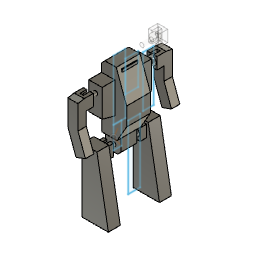
robo v3 (Autodesk Fusion 360 design; units mm, degrees)
Autodesk Fusion 360 part; units mm, degrees
note: some values were not read from the file. Set by a fixed rule: which face or edge a step refers to.
sketch "スケッチ1" plane through (0, 0, 0) normal (1, 0, 0) x (0, 1, 0) in component "球形ジョイント v1"
  circle A0 centre (0, 0) radius 2.5
  line L0 (3.5, -3.5) -> (-3.5, -3.5)
  line L1 (-3.5, -3.5) -> (-3.5, 3.5)
  line L2 (-3.5, 3.5) -> (3.5, 3.5)
  line L3 (3.5, 3.5) -> (3.5, -3.5)
  line L4 (3.5, -3.5) -> (-3.5, 3.5) construction
  line L5 (-3.5, -3.5) -> (3.5, 3.5) construction
  line L6 (4.5, -3.5) -> (2.5, -3.5)
  line L7 (2.5, -3.5) -> (2.5, 3.5)
  line L8 (2.5, 3.5) -> (4.5, 3.5)
  line L9 (4.5, 3.5) -> (4.5, -3.5)
  line L10 (4.5, -3.5) -> (2.5, 3.5) construction
  line L11 (2.5, -3.5) -> (4.5, 3.5) construction
  line L12 (2.5, 3.5) -> (2.5, 3.8624)
  line L13 (2.5, 3.8624) -> (-1, 3.8624)
  line L14 (-1, 3.8624) -> (-1, -3.5)
  point P0 (3.5, 0)
  dimension "d1" = 5
  dimension "d4" = 7
  dimension "d5" = 7
  dimension "d8" = 2
  dimension "d9" = 7
  dimension "d12" = 3.5
  constraint coincident A0.centre origin
  constraint horizontal L0
  constraint perpendicular L0 L1
  constraint parallel L0 L2
  constraint parallel L1 L3
  constraint coincident L4 A0.centre
  constraint coincident L5 A0.centre
  constraint horizontal L6
  constraint perpendicular L6 L7
  constraint parallel L6 L8
  constraint parallel L7 L9
  constraint coincident L10 P0
  constraint coincident L11 P0
  constraint midpoint L3 P0
  constraint perpendicular L8 L12
  constraint perpendicular L12 L13
  constraint coincident L0 L14.end
  constraint perpendicular L0 L14
  measures "d1" diameter of A0
  measures "d4" distance of L1.end L2.end
  measures "d5" distance of L0.end L1.end
  measures "d8" distance of L7.end L8.end
  measures "d9" distance of L6.end L7.end
  measures "d12" distance of L12.end L13.end
sphere "球プリミティブ1" add diameter 5 placed x (0, 1, 0) y (0, 0, 1) z (1, 0, 0) at (0, 0, 0) makes body 1 in component "球形ジョイント v1"
sphere "球プリミティブ2" add diameter 5.5 placed x (0, 1, 0) y (0, 0, 1) z (1, 0, 0) at (0, 0, 0) separate body makes body 2 in component "球形ジョイント v1"
extrude "押し出し1" add sketch "スケッチ1" along normal mid plane 7 separate body contours A0 L14 | A0 L0 L7 L14 | L0 L2 L3 L6 L7 L8 | A0 L2 L7 L14 | A0 L14 | A0 L0 L1 L2 L14 makes body 3 in component "球形ジョイント v1"
move_face "面を移動1" by (3.5, 0, 0) 1 faces at (-3.5, -1.1667, -1.1667) on bodies 3 in component "球形ジョイント v1"
move_face "面を移動2" by (1, 0, 0) 1 faces at (0, 1.1667, 1.1667) on bodies 3 in component "球形ジョイント v1"
move_face "面を移動3" by (0, 1, 0) 1 faces at (1.8333, 3.5, 1.1667) on bodies 3 in component "球形ジョイント v1"
extrude "押し出し2" add sketch "スケッチ1" along normal blind 3.5 separate body contours L0 L2 L3 L6 L7 L8 | L3 L6 L8 L9 makes body 4 in component "球形ジョイント v1"
move_face "面を移動4" by (0, 0.5, 0) 2 faces at (1.1667, 2.5, 1.1667) (1.1667, 2.5, -2.3333) on bodies 4 in component "球形ジョイント v1"
move_face "面を移動5" by (-0.5, 0, 0) 1 faces at (3.5, 1.8333, -1.1667) on bodies 3 in component "球形ジョイント v1"
move_face "面を移動6" by (-0.5, 0, 0) 1 faces at (3.5, 4, 0) on bodies 4 in component "球形ジョイント v1"
move_face "面を移動7" by (0, -1.5, 0) 1 faces at (1.6667, 4.5, 1.1667) on bodies 3 in component "球形ジョイント v1"
move_face "面を移動8" by (0, 2.5, 0) 1 faces at (1.6667, -3.5, -1.1667) on bodies 3 in component "球形ジョイント v1"
copy_body "ボディのコピーと貼り付け1" bodies 2 makes body 5 in component "球形ジョイント v1"
combine "結合1" operation cut target body 3 tool bodies 5 in component "球形ジョイント v1"
combine "結合2" operation add target body 3 tool bodies 4 in component "球形ジョイント v1"
mirror "ミラー1" about plane through (0, 0, 0) normal (-1, 0, 0) of bodies 3 merged in component "球形ジョイント v1"
cylinder "円柱プリミティブ1" add diameter 2.5 height -8 placed x (1, 0, 0) y (0, 0, -1) z (0, 1, 0) at (0, 0, 0) bodies 1 in component "球形ジョイント v1"
copy_body "ボディ -> コンポーネント1" bodies 1 removing the originals makes body 6 in component "丸オス"
copy_body "ボディ -> コンポーネント2" bodies 3 removing the originals makes body 7 in component "丸メス"
sketch "スケッチ1 (2)" plane through (0, 0, 0) normal (1, 0, 0) x (0, 1, 0) in component "Component'''"
  line L0 (7.0755, 32.0667) -> (-0.0136, 32.0667)
  line L1 (-0.0504, 67.9333) -> (7.0755, 67.9333)
  line L2 (4.745, 18.8123) -> (0, 18.8123)
  line L3 (-0.0136, 32.0667) -> (4.745, 32.0667)
  line L4 (4.745, 32.0667) -> (4.745, 18.8123)
  line L5 (4.745, 18.8123) -> (-0.0068, 25.449) construction
  line L6 (-0.0068, 25.43) -> (4.745, 32.0667) construction
  line L7 (8.7818, 29.9549) -> (15.9135, 29.9549)
  line L8 (15.9135, 29.9549) -> (15.9135, -8.3231)
  line L9 (15.9135, -8.3231) -> (8.7818, -8.3231)
  line L10 (8.7818, -8.3231) -> (8.7818, 29.9549)
  line L11 (17.6609, 60.9458) -> (24.0648, 60.9458)
  line L12 (24.0648, 60.9458) -> (24.0648, 30.3816)
  line L13 (24.0648, 30.3816) -> (17.6609, 30.3816)
  line L14 (17.6609, 30.3816) -> (17.6609, 60.9458)
  line L15 (7.0755, 67.9333) -> (7.0755, 32.0667)
  line L16 (7.0755, 62.9476) -> (14.7507, 62.9476)
  line L17 (14.7507, 62.9476) -> (14.7507, 44.3268)
  line L18 (14.7507, 44.3268) -> (7.0755, 44.3268)
  line L19 (7.0755, 44.3268) -> (7.0755, 62.9476)
  line L20 (-0.0504, 67.9333) -> (0, 18.8123)
  point P0 (0, 25.4395)
  constraint horizontal L0
  constraint parallel L0 L1
  constraint horizontal L2
  constraint parallel L2 L3
  constraint coincident L5 P0
  constraint coincident L6 P0
  constraint horizontal L7
  constraint vertical L8
  constraint horizontal L9
  constraint vertical L10
  constraint horizontal L11
  constraint vertical L12
  constraint horizontal L13
  constraint vertical L14
  constraint perpendicular L0 L15
  constraint horizontal L16
  constraint vertical L17
  constraint horizontal L18
  constraint vertical L19
  constraint coincident L15 L16.start
  constraint coincident L20 L0.end
  constraint coincident L20 L5.end
  constraint coincident L20 L6.start
extrude "押し出し1'" add sketch "スケッチ1 (2)" along normal blind 15 separate body contours L0 L1 L3 L15 L19 L20 makes body 8 in component "Component'''"
ref_plane "作業平面1" through (7.5, 3.5125, 52.9333) normal (0, 0, 1) x (0, -1, 0) in component "Component'''"
split "分割1" by plane through (7.5, 3.5125, 52.9333) normal (0, 0, 1) bodies 8 makes body 9 at (5, -0.0453, 62.9333) in component "Component'''"
move_face "面を移動1'" to x (0.965926, 0, 0.258819) y (0, 1, 0) z (-0.258819, 0, 0.965926) at (14.2113, 0, -2.0786) 1 faces at (15, 2.33, 61.2714) on bodies 9 in component "Component'''"
ref_plane "作業平面2" through (7.5, 3.5309, 42.0667) normal (0, 0, -1) x (0, 1, 0) in component "Component'''"
split "分割2" by plane through (7.5, 3.5309, 42.0667) normal (0, 0, -1) bodies 8 makes body 10 at (5, -0.0205, 38.7334) in component "Component'''"
move_face "面を移動2'" to x (0.996195, 0, 0.087156) y (0, 1, 0) z (-0.087156, 0, 0.996195) at (4.6705, 0, -1.1059) 1 faces at (12.7658, 2.33, 61.2714) on bodies 9 in component "Component'''"
move_face "面を移動3'" to x (0.866025, 0, -0.5) y (0, 1, 0) z (0.5, 0, 0.866025) at (-19.0237, 0, 13.1359) 1 faces at (15, 3.9322, 38.7334) on bodies 10 in component "Component'''"
extrude "押し出し2'" add sketch "スケッチ1 (2)" along normal blind 5 contours L15 L16 L17 L18 L19 bodies 8 9 in component "Component'''"
move_face "面を移動4'" by (3, 0, 0) 1 faces at (5, 12.1923, 50.5338) on bodies 8 in component "Component'''"
extrude "押し出し3" add sketch "スケッチ1 (2)" along normal blind 9.21 contours L0 L2 L3 L4 L20 bodies 10 in component "Component'''"
move_face "面を移動5'" to x (1, 0, 0) y (0, 0.965926, 0.258819) z (0, -0.258819, 0.965926) at (0, 11.7137, -0.3209) 1 faces at (5.3333, 9.6339, 44.3268) on bodies 8 in component "Component'''"
copy_body "ボディのコピーと貼り付け1'" bodies 6 body 6 seen with x (1, 0, 0) y (0, 1, 0) z (0, 0, 1) at (0, 25, 65) makes body 11 in component "Component'''"
move_body "移動1" bodies 11 to x (1, 0, 0) y (0, 1, 0) z (0, 0, 1) at (4, -5, -7) in component "Component'''"
move_face "面を移動6'" by (0, 0, 4) 1 faces at (3.07, 3.1633, 18.8123) on bodies 10 in component "Component'''"
copy_body "ボディのコピーと貼り付け2" bodies 11 makes body 12 in component "Component'''"
move_body "移動2" bodies 12 to x (1, 0, 0) y (0, 1, 0) z (0, 0, 1) at (1, 0, -30) in component "Component'''"
move_body "移動3" bodies 12 to x (1, 0, 0) y (0, 1, 0) z (0, 0, 1) at (-0.0516, -10, -0.9987) in component "Component'''"
combine "結合1'" operation add target body 8 tool bodies 10 11 12 in component "Component'''"
mirror "ミラー1'" about plane through (0, -0.0504, 67.9333) normal (0, -0.999999, -0.001027) of bodies 8 merged in component "Component'''"
delete_face "面を削除1" 1 faces at (11.3603, 2.33, 62.9333) on bodies 8 in component "Component'''"
delete_face "面を削除2" 1 faces at (13.0755, 2.346, 38.7334) on bodies 8 in component "Component'''"
delete_face "面を削除3" 1 faces at (6.3621, 4.7002, 67.9333) on bodies 8 in component "Component'''"
delete_face "面を削除4" 1 faces at (3.07, 3.162, 22.8123) on bodies 8 in component "Component'''"
move_face "面を移動7'" by (0, -0.0041, 2) 1 faces at (6.3603, -2.4257, 67.9284) on bodies 8 in component "Component'''"
sketch "スケッチ2" plane through (0, 0, 0) normal (1, 0, 0) x (0, 1, 0) in component "Component'''"
  line L0 (4.5755, 66.4765) -> (-4.8034, 66.4765)
  line L1 (-4.8034, 66.4765) -> (-4.8034, 68.2273)
  line L2 (-4.8034, 68.2273) -> (4.5755, 68.2273)
  line L3 (4.5755, 68.2273) -> (4.5755, 66.4765)
  line L4 (4.5755, 66.4765) -> (-4.8034, 68.2273) construction
  line L5 (-4.8034, 66.4765) -> (4.5755, 68.2273) construction
  point P0 (-0.1139, 67.3519)
  constraint horizontal L0
  constraint perpendicular L0 L1
  constraint parallel L0 L2
  constraint parallel L1 L3
  constraint coincident L4 P0
  constraint coincident L5 P0
extrude "押し出し4" add sketch "スケッチ2" along normal blind 10 bodies 8 in component "Component'''"
copy_body "ボディのコピーと貼り付け3" bodies 7 body 7 seen with x (1, 0, 0) y (0, 1, 0) z (0, 0, 1) at (0, 25, 65) makes body 13 in component "Component'''"
move_body "移動4" bodies 13 to x (1, 0, 0) y (0, 1, 0) z (0, 0, 1) at (4, -5, -6) in component "Component'''"
move_body "移動5" bodies 13 to x (1, 0, 0) y (0, 1, 0) z (0, 0, 1) at (0, 0, -1) in component "Component'''"
sketch "スケッチ3" plane through (0, 0, 0) normal (1, 0, 0) x (0, 1, 0) in component "Component'''"
  line L0 (23.2637, 61.4859) -> (28.2637, 61.4859)
  line L1 (28.2637, 61.4859) -> (28.2637, 31.4859)
  line L2 (28.2637, 31.4859) -> (23.2637, 31.4859)
  line L3 (23.2637, 31.4859) -> (23.2637, 61.4859)
  dimension "d29" = 5
  dimension "d30" = 30
  constraint horizontal L0
  constraint vertical L1
  constraint horizontal L2
  constraint vertical L3
  measures "d29" distance of L0.start L0.end
  measures "d30" distance of L0.start L2.end
extrude "押し出し5" add sketch "スケッチ3" along normal blind 7 and the other way blind -1 separate body makes body 14 in component "Component'''"
ref_plane "作業平面3" through (4, 25.7637, 45.4859) normal (0, 0, -1) x (0, 1, 0) in component "Component'''"
split "分割3" by plane through (4, 25.7637, 45.4859) normal (0, 0, -1) bodies 14 makes body 15 at (3, 23.2637, 36.1525) in component "Component'''"
move_body "移動6" bodies 15 to x (0.939693, 0, 0.34202) y (0, 1, 0) z (-0.34202, 0, 0.939693) at (15.6174, 0, 2.4011) in component "Component'''"
combine "結合2'" operation add target body 14 tool bodies 15 in component "Component'''"
extrude "押し出し6" add sketch "スケッチ1 (2)" along normal blind 9 separate body contours L7 L8 L9 L10 makes body 16 in component "Component'''"
move_body "移動7" bodies 16 to x (1, 0, 0) y (0, 1, 0) z (0, 0, 1) at (0, 19, 0) in component "Component'''"
copy_body "ボディのコピーと貼り付け4" bodies 7 body 7 seen with x (1, 0, 0) y (0, 1, 0) z (0, 0, 1) at (0, 25, 65) makes body 17 in component "Component'''"
move_body "移動8" bodies 17 to x (1, 0, 0) y (0, 1, 0) z (0, 0, 1) at (5, -16, -38) in component "Component'''"
move_body "移動9" bodies 16 to x (1, 0, 0) y (0, 1, 0) z (0, 0, 1) at (0, -16, 2) in component "Component'''"
move_face "面を移動8'" to x (0.984808, 0, 0.173648) y (0, 1, 0) z (-0.173648, 0, 0.984808) at (5.6856, 0, -1.0774) 1 faces at (9, 14.159, 6.4363) on bodies 16 in component "Component'''"
chamfer "面取り1" distance 2 angle 45 2 edges at (9.21, -0.0041, 22.8123) (0, -0.0041, 22.8123) on bodies 8 in component "Component'''"
chamfer "面取り2" distance 2 angle 45 1 edges at (0, -0.0525, 69.9333) on bodies 8 in component "Component'''"
combine "結合3" operation add target body 13 tool bodies 14 in component "Component'''"
combine "結合4" operation add target body 16 tool bodies 17 in component "Component'''"
ref_plane "作業平面4" through (7.5, -0.033, 50.9964) normal (0, -0.999999, -0.001027) x (0, -0.001027, 0.999999) in component "Component'''"
mirror "ミラー2" about plane through (7.5, -0.033, 50.9964) normal (0, -0.999999, -0.001027) of bodies 13 makes body 18 in component "Component'''"
mirror "ミラー3" about plane through (7.5, -0.033, 50.9964) normal (0, -0.999999, -0.001027) of bodies 16 makes body 19 in component "Component'''"
move_face "面を移動9" to x (1, 0, 0) y (0, 0.984808, 0.173648) z (0, -0.173648, 0.984808) at (0, 10.2946, 5.2029) 1 faces at (5, -27.0967, 61.4303) on bodies 18 in component "Component'''"
move_face "面を移動10" to x (1, 0, 0) y (0, 0.984808, -0.173648) z (0, 0.173648, 0.984808) at (0, -10.3047, 5.1885) 1 faces at (5, 27.0091, 61.4859) on bodies 13 in component "Component'''"
component "球形ジョイント v1" placed x (1, 0, 0) y (0, 1, 0) z (0, 0, 1) at (0, 25, 65)
component "Component'''" placed x (1, 0, 0) y (0, 1, 0) z (0, 0, 1) at (0, 0, 0)
component "丸オス" placed x (1, 0, 0) y (0, 1, 0) z (0, 0, 1) at (0, 0, 0) in component "球形ジョイント v1"
component "丸メス" placed x (1, 0, 0) y (0, 1, 0) z (0, 0, 1) at (0, 0, 0) in component "球形ジョイント v1"
hidden bodies 2
named bodies: "丸オス", "丸メス", "Body", "丸オス (1)", "LeftArm", "leftReg", "丸メス (1)", "RightArm", "RightReg"
